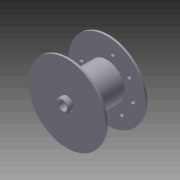
# Autodesk Inventor part: Spool 1764
Saved by Autodesk Inventor 2011 (Build 150239000, 239)
## iProperties
Created: 2010-02-11
Part Number: Spool 1764
Document SubType Name: Modeling
Designer: jrobinson
Density: 1 g/cm^3
Author: jrobinson
Autodesk Inventor part; units mm, degrees
ref_plane "XZ Plane" through (0, 0, 0) normal (0, 1, 0) x (-1, 0, 0)
ref_plane "XY Plane" through (0, 0, 0) normal (0, 0, 1) x (1, 0, 0)
sketch "Sketch1" plane through (0, 0, 0) normal (0, 0, 1) x (1, 0, 0)
  circle A0 centre (0, 0) radius 54.8005
  dimension "d0" = 109.601
  constraints: 1 centre point, 1 coincident
  measures "d0" diameter of A0
extrude "Extrusion1" add sketch "Sketch1" along normal blind 2.921
sketch "Sketch2" plane through (0, 0, 2.921) normal (0, 0, 1) x (1, 0, 0)
  circle A0 centre (0, 0) radius 54.8005 projected
  circle A1 centre (0, 0) radius 25.6794
  circle A2 centre (0, 0) radius 22.7584
  dimension "d3" = 51.3588
  dimension "d17" = 2.921
  constraints: 2 centre point, 2 coincident
  measures "d3" diameter of A1
  measures "d17" radial gap between concentric circles of A1 A2
extrude "Extrusion2" add sketch "Sketch2" along normal blind 53.467 contours A1
sketch "Sketch3" plane through (0, 0, 56.388) normal (0, 0, 1) x (1, 0, 0)
  circle A0 centre (0, 0) radius 25.6794 projected
  circle A1 centre (0, 0) radius 54.8005 projected
  circle A2 centre (0, 0) radius 54.8005
  constraints: 1 centre point, 1 coincident, 1 concentric
extrude "Extrusion3" add sketch "Sketch3" along normal blind 2.921 contours A0 | A1
sketch "Sketch4" plane through (0, 0, 59.309) normal (0, 0, 1) x (1, 0, 0)
  circle A0 centre (0, 0) radius 54.8005 projected
  circle A1 centre (0, 0) radius 9.525
  dimension "d8" = 19.05
  constraints: 1 centre point, 1 coincident
  measures "d8" diameter of A1
extrude "Extrusion4" add sketch "Sketch4" along normal blind 6.35 contours A1
sketch "Sketch5" plane through (0, 0, 65.659) normal (0, 0, 1) x (1, 0, 0)
  circle A0 centre (0, 0) radius 9.525 projected
  circle A1 centre (0, 0) radius 6.223
  dimension "d11" = 12.446
  constraints: 1 centre point, 1 coincident
  measures "d11" diameter of A1
sketch "Sketch6" plane through (0, 0, 0) normal (0, 0, -1) x (-1, 0, 0)
  circle A0 centre (0, 0) radius 9.525 projected
  circle A1 centre (0, 0) radius 9.525 projected
  circle A2 centre (0, 0) radius 9.525
  dimension "d12" = 19.05
  constraints: 1 centre point, 1 coincident
  measures "d12" diameter of A2
extrude "Extrusion5" add sketch "Sketch6" along normal blind 12.7
extrude "Extrusion6" cut sketch "Sketch5" against normal through all contours A1
sketch "Sketch7" plane through (0, 0, 2.921) normal (0, 0, 1) x (1, 0, 0)
  circle A0 centre (0, 0) radius 6.223 projected
  circle A1 centre (0, 0) radius 6.223 projected
  circle A2 centre (0, 0) radius 9.525 projected
extrude "Extrusion7" add sketch "Sketch7" along normal through all
chamfer "Chamfer1" distance 1.5875 angle 45 2 edges at (-9.525, 0, 65.659) (9.525, 0, -12.7)
ref_plane "Work Plane1" through (25.6794, 0, 2.921) normal (1, 0, 0) x (0, 1, 0)
sketch "Sketch8" plane through (25.6794, 0, 2.921) normal (1, 0, 0) x (0, 1, 0)
  line L0 (-54.8005, 53.467) -> (54.8005, 53.467) projected
  line L1 (-25.6794, 53.467) -> (25.6794, 53.467) projected
  line L2 (-54.8005, 0) -> (54.8005, 0) projected
  line L3 (-25.6794, 0) -> (25.6794, 0) projected
  circle A0 centre (2.6963, 38.862) radius 8.2931
  point P0 (0, -2.921)
  dimension "d23" = 14.605
  dimension "d24" = 16.5862
  constraints: 1 centre point
  measures "d23" distance from line of L0 A0.centre
  measures "d24" diameter of A0
extrude "Extrusion8" cut sketch "Sketch8" against normal blind 12.7
pattern_circular "Circular Pattern1" count 2 over 90 about axis through (0, 0, 2.921) along (0, 0, 1) of "Extrusion8"
sketch "Sketch9" plane through (0, 0, 0) normal (0, 0, -1) x (-1, 0, 0)
  circle A0 centre (0, 0) radius 54.8005 projected
  circle A1 centre (0, 0) radius 28.5115
  circle A2 centre (0, 0) radius 48.9585
  dimension "d30" = 57.023
  dimension "d31" = 97.917
  constraints: 2 centre point, 2 coincident
  measures "d30" diameter of A1
  measures "d31" diameter of A2
extrude "Extrusion9" add sketch "Sketch9" along normal blind 0.635 contours A2
chamfer "Chamfer2" distance 0.635 angle 45 2 edges at (48.9585, 0, -0.635) (28.5115, 0, -0.635)
sketch "Sketch12" plane through (0, 0, 2.921) normal (0, 0, 1) x (1, 0, 0)
  circle A0 centre (0, 0) radius 28.5115 projected
  circle A1 centre (31.0504, 20.3913) radius 3.175 projected
  circle A2 centre (-31.0504, -20.3913) radius 3.175 projected
  circle A3 centre (20.3913, -31.0504) radius 3.175 projected
  circle A4 centre (-36.3748, 7.5371) radius 3.175 projected
  circle A5 centre (7.5371, 36.3748) radius 3.175 projected
  circle A6 centre (36.3748, -7.5371) radius 3.175 projected
  circle A7 centre (-7.5371, -36.3748) radius 3.175 projected
  arc A8 (19.7771, 37.7111) -> (20.5429, 44.5183) centre (-8.1746, 44.3026) ccw projected
  arc A9 (21.6617, 36.661) -> (19.7771, 37.7111) centre (0, 0) ccw projected
  arc A10 (27.0474, 40.8941) -> (21.6617, 36.661) centre (41.9748, 16.3602) ccw projected
  arc A11 (29.0839, 39.4717) -> (27.0474, 40.8941) centre (0, 0) ccw projected
  arc A12 (26.9634, 32.958) -> (29.0839, 39.4717) centre (0.9108, 45.0412) ccw projected
  arc A13 (28.5981, 31.55) -> (26.9634, 32.958) centre (0, 0) ccw projected
  arc A14 (34.7256, 34.6124) -> (28.5981, 31.55) centre (44.4089, 7.5758) ccw projected
  arc A15 (36.4341, 32.8092) -> (34.7256, 34.6124) centre (0, 0) ccw projected
  arc A16 (33.0459, 26.8557) -> (36.4341, 32.8092) centre (9.9589, 43.9359) ccw projected
  arc A17 (34.3637, 25.1474) -> (33.0459, 26.8557) centre (0, 0) ccw projected
  arc A18 (40.9822, 26.9137) -> (34.3637, 25.1474) centre (45.0248, -1.5187) ccw projected
  arc A19 (42.2928, 24.8034) -> (40.9822, 26.9137) centre (0, 0) ccw projected
  arc A20 (37.7754, 19.6538) -> (42.2928, 24.8034) centre (18.5992, 41.0318) ccw projected
  arc A21 (38.7224, 17.7153) -> (37.7754, 19.6538) centre (0, 0) ccw projected
  arc A22 (45.561, 18.1131) -> (38.7224, 17.7153) centre (43.7975, -10.551) ccw projected
  arc A23 (46.4199, 15.7822) -> (45.561, 18.1131) centre (0, 0) ccw projected
  arc A24 (40.9585, 11.6474) -> (46.4199, 15.7822) centre (26.4782, 36.4479) ccw projected
  arc A25 (41.4958, 9.5579) -> (40.9585, 11.6474) centre (0, 0) ccw projected
  arc A26 (48.2745, 8.571) -> (41.4958, 9.5579) centre (40.777, -19.1514) ccw projected
  arc A27 (48.6467, 6.1149) -> (48.2745, 8.571) centre (0, 0) ccw projected
  arc A28 (42.4646, 3.1641) -> (48.6467, 6.1149) centre (33.2731, 30.3718) ccw projected
  arc A29 (42.5704, 1.0092) -> (42.4646, 3.1641) centre (0, 0) ccw projected
  arc A30 (49.0116, -1.3221) -> (42.5704, 1.0092) centre (36.0871, -26.9677) ccw projected
  arc A31 (48.8818, -3.8028) -> (49.0116, -1.3221) centre (0, 0) ccw projected
  arc A32 (42.2323, -5.4487) -> (48.8818, -3.8028) centre (38.7058, 23.0522) ccw projected
  arc A33 (41.9021, -7.5808) -> (42.2323, -5.4487) centre (0, 0) ccw projected
  arc A34 (47.7422, -11.161) -> (41.9021, -7.5808) centre (29.9199, -33.68) ccw projected
  arc A35 (47.1157, -13.5648) -> (47.7422, -11.161) centre (0, 0) ccw projected
  arc A36 (40.271, -13.8385) -> (47.1157, -13.5648) centre (42.5538, 14.789) ccw projected
  arc A37 (39.5184, -15.8604) -> (40.271, -13.8385) centre (0, 0) ccw projected
  arc A38 (44.5183, -20.543) -> (39.5184, -15.8604) centre (22.5277, -39.0134) ccw projected
  arc A39 (43.4206, -22.7714) -> (44.5183, -20.543) centre (0, 0) ccw projected
  arc A40 (36.661, -21.6617) -> (43.4206, -22.7714) centre (44.6597, 5.9202) ccw projected
  arc A41 (35.5168, -23.4908) -> (36.661, -21.6617) centre (0, 0) ccw projected
  arc A42 (39.4717, -29.0839) -> (35.5168, -23.4908) centre (14.2132, -42.7496) ccw projected
  arc A43 (37.948, -31.0458) -> (39.4717, -29.0839) centre (0, 0) ccw projected
  arc A44 (31.55, -28.5981) -> (37.948, -31.0458) centre (44.9373, -3.1909) ccw projected
  arc A45 (30.0611, -30.1594) -> (31.55, -28.5981) centre (0, 0) ccw projected
  arc A46 (32.8092, -36.4341) -> (30.0611, -30.1594) centre (5.3168, -44.7356) ccw projected
  arc A47 (30.9217, -38.0491) -> (32.8092, -36.4341) centre (0, 0) ccw projected
  arc A48 (25.1475, -34.3637) -> (30.9217, -38.0491) centre (43.3751, -12.1714) ccw projected
  arc A49 (23.3747, -35.5933) -> (25.1475, -34.3637) centre (0, 0) ccw projected
  arc A50 (24.8034, -42.2928) -> (23.3747, -35.5933) centre (-3.7972, -44.8901) ccw projected
  arc A51 (22.6295, -43.4948) -> (24.8034, -42.2928) centre (0, 0) ccw projected
  arc A52 (17.7153, -38.7224) -> (22.6295, -43.4948) centre (40.0371, -20.6536) ccw projected
  arc A53 (15.7313, -39.57) -> (17.7153, -38.7224) centre (0, 0) ccw projected
  arc A54 (15.7822, -46.4199) -> (15.7313, -39.57) centre (-12.7558, -43.2068) ccw projected
  arc A55 (13.4108, -47.1597) -> (15.7822, -46.4199) centre (0, 0) ccw projected
  arc A56 (9.5579, -41.4958) -> (13.4108, -47.1597) centre (35.06, -28.2902) ccw projected
  arc A57 (7.4439, -41.9267) -> (9.5579, -41.4958) centre (0, 0) ccw projected
  arc A58 (6.1149, -48.6467) -> (7.4439, -41.9267) centre (-21.1922, -39.7547) ccw projected
  arc A59 (3.6431, -48.8939) -> (6.1149, -48.6467) centre (0, 0) ccw projected
  arc A60 (1.0092, -42.5704) -> (3.6431, -48.8939) centre (28.6475, -34.7687) ccw projected
  arc A61 (-1.1482, -42.5669) -> (1.0092, -42.5704) centre (0, 0) ccw projected
  arc A62 (-3.8028, -48.8818) -> (-1.1482, -42.5669) centre (-28.7609, -34.6749) ccw projected
  arc A63 (-6.2737, -48.6264) -> (-3.8028, -48.8818) centre (0, 0) ccw projected
  arc A64 (-7.5808, -41.9021) -> (-6.2737, -48.6264) centre (21.0622, -39.8237) ccw projected
  arc A65 (-9.6934, -41.4644) -> (-7.5808, -41.9021) centre (0, 0) ccw projected
  arc A66 (-13.5648, -47.1157) -> (-9.6934, -41.4644) centre (-35.1522, -28.1756) ccw projected
  arc A67 (-15.9337, -46.3682) -> (-13.5648, -47.1157) centre (0, 0) ccw projected
  arc A68 (-15.8604, -39.5184) -> (-15.9337, -46.3682) centre (12.6147, -43.2483) ccw projected
  arc A69 (-17.8417, -38.6644) -> (-15.8604, -39.5184) centre (0, 0) ccw projected
  arc A70 (-22.7714, -43.4207) -> (-17.8417, -38.6644) centre (-40.1043, -20.5228) ccw projected
  arc A71 (-24.9414, -42.2116) -> (-22.7714, -43.4207) centre (0, 0) ccw projected
  arc A72 (-23.4908, -35.5168) -> (-24.9414, -42.2116) centre (3.6506, -44.9023) ccw projected
  arc A73 (-25.2595, -34.2814) -> (-23.4908, -35.5168) centre (0, 0) ccw projected
  arc A74 (-31.0458, -37.948) -> (-25.2595, -34.2814) centre (-43.4146, -12.0297) ccw projected
  arc A75 (-32.928, -36.3268) -> (-31.0458, -37.948) centre (0, 0) ccw projected
  arc A76 (-30.1594, -30.0611) -> (-32.928, -36.3268) centre (-5.4629, -44.718) ccw projected
  arc A77 (-31.6432, -28.4949) -> (-30.1594, -30.0611) centre (0, 0) ccw projected
  arc A78 (-38.0491, -30.9217) -> (-31.6432, -28.4949) centre (-44.9475, -3.0442) ccw projected
  arc A79 (-39.5665, -28.9549) -> (-38.0491, -30.9217) centre (0, 0) ccw projected
  arc A80 (-35.5933, -23.3747) -> (-39.5665, -28.9549) centre (-14.3527, -42.7029) ccw projected
  arc A81 (-36.7315, -21.5419) -> (-35.5933, -23.3747) centre (0, 0) ccw projected
  arc A82 (-43.4948, -22.6295) -> (-36.7315, -21.5419) centre (-44.6402, 6.066) ccw projected
  arc A83 (-44.5851, -20.3975) -> (-43.4948, -22.6295) centre (0, 0) ccw projected
  arc A84 (-39.57, -15.7313) -> (-44.5851, -20.3975) centre (-22.6549, -38.9396) ccw projected
  arc A85 (-40.316, -13.707) -> (-39.57, -15.7313) centre (0, 0) ccw projected
  arc A86 (-47.1597, -13.4108) -> (-40.316, -13.707) centre (-42.5053, 14.9278) ccw projected
  arc A87 (-47.7784, -11.005) -> (-47.1597, -13.4108) centre (0, 0) ccw projected
  arc A88 (-41.9267, -7.4439) -> (-47.7784, -11.005) centre (-30.0297, -33.5821) ccw projected
  arc A89 (-42.2499, -5.3108) -> (-41.9267, -7.4439) centre (0, 0) ccw projected
  arc A90 (-48.8939, -3.6431) -> (-42.2499, -5.3108) centre (-38.6303, 23.1785) ccw projected
  arc A91 (-49.0157, -1.162) -> (-48.8939, -3.6431) centre (0, 0) ccw projected
  arc A92 (-42.5669, 1.1482) -> (-49.0157, -1.162) centre (-36.175, -26.8498) ccw projected
  arc A93 (-42.4541, 3.3027) -> (-42.5669, 1.1482) centre (0, 0) ccw projected
  arc A94 (-48.6264, 6.2737) -> (-42.4541, 3.3027) centre (-33.1737, 30.4803) ccw projected
  arc A95 (-48.2463, 8.7285) -> (-48.6264, 6.2737) centre (0, 0) ccw projected
  arc A96 (-41.4644, 9.6934) -> (-48.2463, 8.7285) centre (-40.8393, -19.0182) ccw projected
  arc A97 (-40.9202, 11.7811) -> (-41.4644, 9.6934) centre (0, 0) ccw projected
  arc A98 (-46.3682, 15.9337) -> (-40.9202, 11.7811) centre (-26.359, 36.5341) ccw projected
  arc A99 (-45.5016, 18.2618) -> (-46.3682, 15.9337) centre (0, 0) ccw projected
  arc A100 (-38.6644, 17.8417) -> (-45.5016, 18.2618) centre (-43.8317, -10.408) ccw projected
  arc A101 (-37.7111, 19.7771) -> (-38.6644, 17.8417) centre (0, 0) ccw projected
  arc A102 (-42.2116, 24.9414) -> (-37.7111, 19.7771) centre (-18.4652, 41.0923) ccw projected
  arc A103 (-40.8941, 27.0474) -> (-42.2116, 24.9414) centre (0, 0) ccw projected
  arc A104 (-34.2814, 25.2595) -> (-40.8941, 27.0474) centre (-45.0295, -1.3717) ccw projected
  arc A105 (-32.958, 26.9634) -> (-34.2814, 25.2595) centre (0, 0) ccw projected
  arc A106 (-36.3268, 32.928) -> (-32.958, 26.9634) centre (-9.8154, 43.9682) ccw projected
  arc A107 (-34.6124, 34.7256) -> (-36.3268, 32.928) centre (0, 0) ccw projected
  arc A108 (-28.4949, 31.6432) -> (-34.6124, 34.7256) centre (-44.3839, 7.7208) ccw projected
  arc A109 (-26.8557, 33.0459) -> (-28.4949, 31.6432) centre (0, 0) ccw projected
  arc A110 (-28.9549, 39.5665) -> (-26.8557, 33.0459) centre (-0.7637, 45.044) ccw projected
  arc A111 (-26.9137, 40.9822) -> (-28.9549, 39.5665) centre (0, 0) ccw projected
  arc A112 (-21.5419, 36.7315) -> (-26.9137, 40.9822) centre (-41.9212, 16.4971) ccw projected
  arc A113 (-19.6538, 37.7754) -> (-21.5419, 36.7315) centre (0, 0) ccw projected
  arc A114 (-20.3975, 44.5851) -> (-19.6538, 37.7754) centre (8.3192, 44.2756) ccw projected
  arc A115 (-18.1131, 45.561) -> (-20.3975, 44.5851) centre (0, 0) ccw projected
  arc A116 (-13.707, 40.316) -> (-18.1131, 45.561) centre (-37.7422, 24.5981) ccw projected
  arc A117 (-11.6474, 40.9585) -> (-13.707, 40.316) centre (0, 0) ccw projected
  arc A118 (-11.005, 47.7784) -> (-11.6474, 40.9585) centre (17.0615, 41.6947) ccw projected
  arc A119 (-8.571, 48.2745) -> (-11.005, 47.7784) centre (0, 0) ccw projected
  arc A120 (-5.3108, 42.2499) -> (-8.571, 48.2745) centre (-32.018, 31.692) ccw projected
  arc A121 (-3.1641, 42.4646) -> (-5.3108, 42.2499) centre (0, 0) ccw projected
  arc A122 (-1.162, 49.0157) -> (-3.1641, 42.4646) centre (25.1053, 37.4067) ccw projected
  arc A123 (1.3221, 49.0116) -> (-1.162, 49.0157) centre (0, 0) ccw projected
  arc A124 (3.3027, 42.4541) -> (1.3221, 49.0116) centre (-24.9831, 37.4885) ccw projected
  arc A125 (5.4487, 42.2323) -> (3.3027, 42.4541) centre (0, 0) ccw projected
  arc A126 (8.7285, 48.2463) -> (5.4487, 42.2323) centre (32.1214, 31.5873) ccw projected
  arc A127 (11.161, 47.7422) -> (8.7285, 48.2463) centre (0, 0) ccw projected
  arc A128 (11.7811, 40.9202) -> (11.161, 47.7422) centre (-16.9253, 41.7502) ccw projected
  arc A129 (13.8385, 40.271) -> (11.7811, 40.9202) centre (0, 0) ccw projected
  arc A130 (18.2618, 45.5016) -> (13.8385, 40.271) centre (37.8223, 24.4748) ccw projected
  arc A131 (20.5429, 44.5183) -> (18.2618, 45.5016) centre (0, 0) ccw projected
extrude "Extrusion11" cut sketch "Sketch12" against normal blind 25.4 contours A1 | A2 | A3 | A4 | A5 | A6 | A7
body "Solid1"
